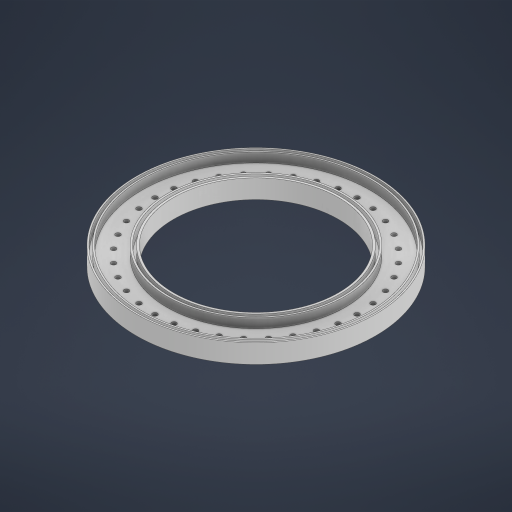
# Autodesk Inventor part: PethFormaFlanec
Saved by Autodesk Inventor 2024 (Build 280153000, 153)
## iProperties
Created: 2023-12-11
Part Number: PethFormaFlanec
Material: Generic
Document SubType Name: Modeling
Designer: KirikDK
Mass: 156.88 g
Surface Area: 801.208 cm^2
Volume: 156.88 cm^3
Density: 1 g/cm^3
Appearance: Default
Author: KirikDK
Autodesk Inventor part; units mm, degrees
ref_plane "YZ Plane" through (0, 0, 0) normal (1, 0, 0) x (0, 1, 0)
ref_plane "XZ Plane" through (0, 0, 0) normal (0, 1, 0) x (-1, 0, 0)
ref_plane "XY Plane" through (0, 0, 0) normal (0, 0, 1) x (1, 0, 0)
sketch "Sketch1" plane through (0, 0, 0) normal (0, 1, 0) x (-1, 0, 0)
  circle A0 centre (0.143, 11.2846) radius 71.8694
  circle A1 centre (0.143, 11.2846) radius 74.247
  circle A2 centre (0.143, 11.2846) radius 98.333
  circle A3 centre (0.143, 11.2846) radius 100.5055
  circle A4 centre (0.143, 11.2846) radius 70.1276
  circle A5 centre (0.143, 11.2846) radius 75.7155
  circle A6 centre (0.143, 11.2846) radius 97.0759
  circle A7 centre (0.143, 11.2846) radius 101.7155
  point P0 (0, 0)
  constraints: 8 centre point, 7 coincident
extrude "Extrusion1" add sketch "Sketch1" along normal blind 8
sketch "Sketch2" plane through (-0.143, 0, 11.2846) normal (0, -1, 0) x (1, 0, 0)
  circle A0 centre (0, 0) radius 101.7155
  circle A1 centre (0, 0) radius 70.1276
  point P0 (0.143, -11.2846)
  constraints: 2 centre point, 1 coincident
extrude "Extrusion2" add sketch "Sketch2" along normal blind 8
sketch "Sketch3" plane through (-0.143, -8, 11.2846) normal (0, -1, 0) x (1, 0, 0)
  circle A0 centre (0, 0) radius 72.5
  circle A1 centre (0, 0) radius 100
  circle A2 centre (0, -86) radius 2
  circle A3 centre (14.9337, -84.6935) radius 2
  circle A4 centre (29.4137, -80.8136) radius 2
  circle A5 centre (43, -74.4782) radius 2
  circle A6 centre (55.2797, -65.8798) radius 2
  circle A7 centre (65.8798, -55.2797) radius 2
  circle A8 centre (74.4782, -43) radius 2
  circle A9 centre (80.8136, -29.4137) radius 2
  circle A10 centre (84.6935, -14.9337) radius 2
  circle A11 centre (86, 0) radius 2
  circle A12 centre (84.6935, 14.9337) radius 2
  circle A13 centre (80.8136, 29.4137) radius 2
  circle A14 centre (74.4782, 43) radius 2
  circle A15 centre (65.8798, 55.2797) radius 2
  circle A16 centre (55.2797, 65.8798) radius 2
  circle A17 centre (43, 74.4782) radius 2
  circle A18 centre (29.4137, 80.8136) radius 2
  circle A19 centre (14.9337, 84.6935) radius 2
  circle A20 centre (0, 86) radius 2
  circle A21 centre (-14.9337, 84.6935) radius 2
  circle A22 centre (-29.4137, 80.8136) radius 2
  circle A23 centre (-43, 74.4782) radius 2
  circle A24 centre (-55.2797, 65.8798) radius 2
  circle A25 centre (-65.8798, 55.2797) radius 2
  circle A26 centre (-74.4782, 43) radius 2
  circle A27 centre (-80.8136, 29.4137) radius 2
  circle A28 centre (-84.6935, 14.9337) radius 2
  circle A29 centre (-86, 0) radius 2
  circle A30 centre (-84.6935, -14.9337) radius 2
  circle A31 centre (-80.8136, -29.4137) radius 2
  circle A32 centre (-74.4782, -43) radius 2
  circle A33 centre (-65.8798, -55.2797) radius 2
  circle A34 centre (-55.2797, -65.8798) radius 2
  circle A35 centre (-43, -74.4782) radius 2
  circle A36 centre (-29.4137, -80.8136) radius 2
  circle A37 centre (-14.9337, -84.6935) radius 2
  circle A38 centre (0, 0) radius 101.7155 projected
  circle A39 centre (0, 0) radius 70.1276 projected
  point P0 (0.143, -11.2846)
  dimension "d6" = 145
  dimension "d7" = 200
  dimension "d8" = 360
  constraints: 38 centre point, 2 coincident, 73 other
  measures "d6" diameter of A0
  measures "d7" diameter of A1
extrude "Extrusion3" cut sketch "Sketch3" against normal blind 8 contours A2 | A3 | A4 | A5 | A6 | A7 | A8 | A9 | A10 | A11 | A12 | A13 | A14 | A15 | A16 | A17 | A18 | A19 | A20 | A21 | A22 | A23 | A24 | A25 | A26 | A27 | A28 | A29 | A30 | A31 | A32 | A33 | A34 | A35 | A36 | A37
body "Solid1"
